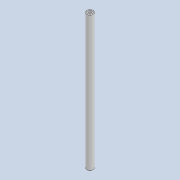
# Autodesk Inventor part: pin_3_60
Saved by Autodesk Inventor 2020 (Build 240168000, 168)
## iProperties
Created: 2021-07-19
Part Number: pin_3_60
Material: Generic
Document SubType Name: Modeling
Designer: Shuang Peng
Density: 1 g/cm^3
Appearance: Default
Author: Shuang Peng
Autodesk Inventor part; units mm, degrees
ref_plane "YZ Plane" through (0, 0, 0) normal (1, 0, 0) x (0, 1, 0)
ref_plane "XZ Plane" through (0, 0, 0) normal (0, 1, 0) x (-1, 0, 0)
ref_plane "XY Plane" through (0, 0, 0) normal (0, 0, 1) x (1, 0, 0)
sketch "Sketch1" plane through (0, 0, 0) normal (0, 1, 0) x (-1, 0, 0)
  circle A0 centre (0, 0) radius 1.5
  circle A1 centre (0, 0) radius 0.75
  dimension "d0" = 3
  dimension "d1" = 1.5
  constraints: 2 centre point, 2 coincident
  measures "d0" diameter of A0
  measures "d1" diameter of A1
extrude "Extrusion1" add sketch "Sketch1" along normal blind 60
chamfer "Chamfer1" distance 0.25 angle 45 2 edges at (1.5, 60, 0) (1.5, 0, 0)
body "Solid1"
